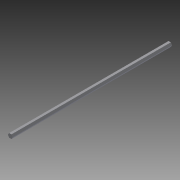
# Autodesk Inventor part: Hexagon Rod
Saved by Autodesk Inventor 2015 (Build 190159000, 159)
## iProperties
Created: 2015-01-14
Part Number: Hexagon Rod
Material: Generic
Document SubType Name: Modeling
Designer: mastkee16
Density: 1 g/cm^3
Appearance: Default
Author: mastkee16
Autodesk Inventor part; units mm, degrees
ref_plane "YZ Plane" through (0, 0, 0) normal (1, 0, 0) x (0, 1, 0)
ref_plane "XZ Plane" through (0, 0, 0) normal (0, 1, 0) x (-1, 0, 0)
ref_plane "XY Plane" through (0, 0, 0) normal (0, 0, 1) x (1, 0, 0)
sketch "Sketch1" plane through (0, 0, 0) normal (0, 0, 1) x (1, 0, 0)
  line L0 (1.8331, 3.175) -> (3.6662, 0)
  line L1 (3.6662, 0) -> (1.8331, -3.175)
  line L2 (1.8331, -3.175) -> (-1.8331, -3.175)
  line L3 (-1.8331, -3.175) -> (-3.6662, 0)
  line L4 (-3.6662, 0) -> (-1.8331, 3.175)
  line L5 (-1.8331, 3.175) -> (1.8331, 3.175)
  point P0 (0, 0)
  point P1 (0, 0)
  dimension "d0" = 6.35
  constraints: 12 end point, 1 coincident, 13 other
  measures "d0" distance between parallel lines of L2 L5
extrude "Extrusion1" add sketch "Sketch1" along normal blind 254
body "Solid1"
